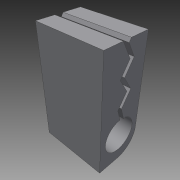
# Autodesk Inventor part: BagClip
Saved by Autodesk Inventor 2015 (Build 190159000, 159)
## iProperties
Created: 2020-03-25
Part Number: BagClip
Material: Generic
Document SubType Name: Modeling
Designer: Dominick Lee
Density: 1 g/cm^3
Appearance: Default
Author: Dominick Lee
Autodesk Inventor part; units mm, degrees
ref_plane "YZ Plane" through (0, 0, 0) normal (1, 0, 0) x (0, 1, 0)
ref_plane "XZ Plane" through (0, 0, 0) normal (0, 1, 0) x (-1, 0, 0)
ref_plane "XY Plane" through (0, 0, 0) normal (0, 0, 1) x (1, 0, 0)
sketch "Sketch1" plane through (0, 0, 0) normal (0, 1, 0) x (-1, 0, 0)
  line L0 (3, 5) -> (-3, 5)
  line L1 (-3, 5) -> (-3, -5)
  line L2 (-3, -5) -> (3, -5)
  line L3 (3, -5) -> (3, 5)
  line L4 (3, 5) -> (-3, -5) construction
  line L5 (-3, 5) -> (3, -5) construction
  point P0 (0, 0)
  dimension "d0" = 6
  dimension "d1" = 10
  constraints: 12 end point, 2 midpoint, 2 parallel, 1 horizontal, 1 perpendicular
  measures "d0" distance of L0.start L0.end
  measures "d1" distance of L1.end L0.end
extrude "Extrusion1" add sketch "Sketch1" along normal blind 4
sketch "Sketch2" plane through (-3, 0, -5) normal (-1, 0, 0) x (0, 0, 1)
  line L0 (0, 0) -> (0, 4) projected
  line L1 (0, 2) -> (2.5, 2)
  arc A0 (3.8928, 2.5568) -> (3.9979, 1.9207) centre (2.5, 2) ccw
  line L2 (0, 4) -> (10, 4) projected
  line L3 (5, 4) -> (5, 2.4)
  line L4 (5, 0) -> (6.2, 0)
  line L5 (0, 0) -> (10, 0) projected
  line L6 (6.2, 0) -> (7.4, 0)
  line L7 (7.4, 0) -> (8.6, 0)
  line L8 (3.9979, 1.9207) -> (5, 1.6)
  line L9 (5, 1.6) -> (6.2, 2.4)
  line L10 (6.2, 2.4) -> (7.4, 1.6)
  line L11 (7.4, 1.6) -> (8.6, 2.4)
  line L12 (8.6, 2.4) -> (10, 1.6)
  line L13 (10, 0) -> (10, 4) projected
  line L14 (3.8567, 2.3333) -> (4.9461, 1.9847)
  line L15 (4.9461, 1.9847) -> (6.2, 2.8206)
  line L16 (6.2, 2.8206) -> (7.4, 2.0206)
  line L17 (7.4, 2.0206) -> (8.5858, 2.8112)
  line L18 (8.5858, 2.8112) -> (9.7271, 2.159)
  line L19 (3.8567, 2.3333) -> (3.8928, 2.5568)
  line L20 (9.7271, 2.159) -> (10, 2.3333)
  dimension "d4" = 2.5
  dimension "d5" = 3
  dimension "d6" = 1.6
  dimension "d7" = 1.6
  dimension "d8" = 1.2
  dimension "d9" = 1.2
  dimension "d10" = 1.2
  dimension "d11" = 0.35
  constraints: 34 end point, 5 point on line, 2 midpoint, 2 parallel, 2 point on circle, 1 centre point, 1 coincident, 1 horizontal, 1 vertical, 3 other
  measures "d4" distance of L1.start L1.end
  measures "d5" diameter of A0
  measures "d6" distance of L4.start L8.end
  measures "d7" distance of L3.start L3.end
  measures "d8" distance of L4.start L4.end
  measures "d9" distance of L4.end L6.end
  measures "d10" distance of L6.end L7.end
  measures "d11" distance between parallel lines of L8 L14
extrude "Extrusion2" cut sketch "Sketch2" against normal blind 6.5 contours A0 L19 L14 L15 L16 L17 L18 L20 L13 L12 L11 L10 L9 L8
fillet "Fillet1" radius 2 1 edges at (0, 4, -5)
body "Solid1"
